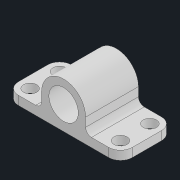
# Autodesk Inventor part: scara-base26
Saved by Autodesk Inventor 2022 (Build 260153000, 153)
## iProperties
Created: 2021-10-30
Part Number: scara-base26
Material: 一般
Document SubType Name: Modeling
Designer: Yuta Kage
Density: 1 g/cm^3
Appearance: 既定
Author: Yuta Kage
Autodesk Inventor part; units mm, degrees
ref_plane "YZ Plane" through (0, 0, 0) normal (1, 0, 0) x (0, 1, 0)
ref_plane "XZ Plane" through (0, 0, 0) normal (0, 1, 0) x (-1, 0, 0)
ref_plane "XY Plane" through (0, 0, 0) normal (0, 0, 1) x (1, 0, 0)
sketch "スケッチ1" plane through (0, 0, 0) normal (0, 0, 1) x (1, 0, 0)
  line L0 (-19.4, -1.5) -> (19.4, -1.5)
  line L1 (19.4, -1.5) -> (19.4, 1.5)
  line L2 (19.4, 1.5) -> (-19.4, 1.5)
  line L3 (-19.4, 1.5) -> (-19.4, -1.5)
  line L4 (-19.4, -1.5) -> (19.4, 1.5) construction
  line L5 (19.4, -1.5) -> (-19.4, 1.5) construction
  circle A0 centre (0, 6.5) radius 5
  circle A1 centre (0, 6.5) radius 7.5
  line L6 (-7.5, 6.5) -> (-7.5, 1.5)
  line L7 (7.5, 6.5) -> (7.5, 1.5)
  point P0 (0, 0)
  point P1 (0, 0)
  point P2 (0, 0)
  point P3 (0, 0)
  dimension "d4" = 10
  dimension "d5" = 3
  dimension "d6" = 38.8
  dimension "d21" = 15
  constraints: 16 end point, 4 midpoint, 3 perpendicular, 3 tangent, 2 centre point, 2 coincident, 2 parallel, 2 point on circle, 2 point on line, 1 horizontal, 1 vertical alignment
  measures "d4" diameter of A0
  measures "d5" distance of L0.end L1.end
  measures "d6" distance of L1.end L2.end
  measures "d21" diameter of A1
extrude "押し出し1" add sketch "スケッチ1" along normal mid plane 18
fillet "フィレット1" radius 2 2 edges at (7.5, 1.5, 0) (-7.5, 1.5, 0)
sketch "スケッチ2" plane through (-19.4, -1.5, 9) normal (0, -1, 0) x (1, 0, 0)
  line L0 (4, -14) -> (34.8, -14)
  line L1 (34.8, -14) -> (34.8, -4)
  line L2 (34.8, -4) -> (4, -4)
  line L3 (4, -4) -> (4, -14)
  line L4 (4, -14) -> (34.8, -4) construction
  line L5 (34.8, -14) -> (4, -4) construction
  point P0 (19.4, -9)
  dimension "d11" = 30.8
  dimension "d12" = 10
  constraints: 12 end point, 2 midpoint, 2 parallel, 1 horizontal, 1 perpendicular
  measures "d11" distance of L2.end L1.end
  measures "d12" distance of L1.end L0.end
hole "穴1" at (15.4, -1.5, 5) at (15.4, -1.5, -5) at (-15.4, -1.5, 5) at (-15.4, -1.5, -5) direction (0, 1, 0) diameter 4.5 end through all clearance for "Flat Head Machine Screw" size "M4" standard "Ansi Metric M Profile"
fillet "フィレット2" radius 4 4 edges at (-19.4, 0, -9) (-19.4, 0, 9) (19.4, 0, -9) (19.4, 0, 9)
ref_plane "作業平面2" through (0, -1.5, 5) normal (-1, 0, 0) x (0, 0, 1)
ref_plane "作業平面1" through (9.5, 0, 9) normal (0, 1, 0) x (1, 0, 0)
